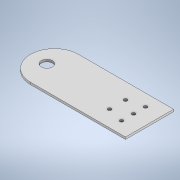
# Autodesk Inventor part: Beslag ekstra håndtag
Saved by Autodesk Inventor 2022 (Build 260153000, 153)
## iProperties
Created: 2022-04-12
Part Number: Beslag ekstra håndtag
Material: Generic
Document SubType Name: Sheet Metal
Designer: Patrick
Density: 1 g/cm^3
Sheet Metal Rule: Default_mm
Appearance: Default
Author: Patrick
Autodesk Inventor part; units mm, degrees
ref_plane "YZ Plane" through (0, 0, 0) normal (1, 0, 0) x (0, 1, 0)
ref_plane "XZ Plane" through (0, 0, 0) normal (0, 1, 0) x (-1, 0, 0)
ref_plane "XY Plane" through (0, 0, 0) normal (0, 0, 1) x (1, 0, 0)
sketch "Sketch2" plane through (0, 0, 0) normal (0, 1, 0) x (-1, 0, 0)
  line L0 (0, 0) -> (109, 0)
  line L1 (109, 0) -> (109, -44)
  line L2 (109, -44) -> (0, -44)
  line L3 (0, -44) -> (0, 0)
  line L4 (44, 0) -> (44, -44) construction
  arc A0 (87, -44) -> (87, 0) centre (87, -22) ccw
  circle A1 centre (94, -22) radius 5.1
  circle A2 centre (29.3333, -14.6667) radius 1.625
  circle A3 centre (29.3333, -29.3333) radius 1.625
  circle A4 centre (14.6667, -11) radius 1.625
  circle A5 centre (14.6667, -22) radius 1.625
  circle A6 centre (14.6667, -33) radius 1.625
  dimension "d36" = 44
  dimension "d37" = 44
  dimension "d38" = 65
  dimension "d41" = 10.2
  dimension "d42" = 22
  dimension "d43" = 15
  dimension "d44" = 14.6667
  dimension "d45" = 14.6667
  dimension "d46" = 14.6667
  dimension "d47" = 11
  dimension "d48" = 11
  dimension "d49" = 11
  dimension "d50" = 11
  dimension "d51" = 3.25
  dimension "d52" = 3.25
  dimension "d53" = 3.25
  dimension "d54" = 3.25
  dimension "d55" = 3.25
  dimension "d56" = 14.6667
  dimension "d57" = 14.6667
  dimension "d58" = 14.6667
  dimension "d59" = 14.6667
  measures "d36" distance between parallel lines of L3 L4
  measures "d37" distance of L2.end L0.start
  measures "d38" distance between parallel lines of L4 L1
  measures "d41" diameter of A1
  measures "d42" distance from line of L2 A1.centre
  measures "d43" distance from line of A1.centre L1
  measures "d44" distance from line of L2 A3.centre
  measures "d45" distance from line of L0 A2.centre
  measures "d46" distance of A2.centre A3.centre
  measures "d47" distance from line of L2 A6.centre
  measures "d48" distance of A5.centre A6.centre
  measures "d49" distance of A5.centre A4.centre
  measures "d50" distance from line of L0 A4.centre
  measures "d51" diameter of A2
  measures "d52" diameter of A3
  measures "d53" diameter of A4
  measures "d54" diameter of A5
  measures "d55" diameter of A6
  measures "d56" distance from line of L4 A3.centre
  measures "d57" distance from line of L4 A2.centre
  measures "d58" distance from line of L3 A6.centre
  measures "d59" distance from line of L3 A4.centre
extrude "Plate3" add sketch "Sketch2" along normal blind 2 contours L0 A0 L2 L3
equation "\"d42\" = 0.5 * d37"
equation "\"d44\" = 0.333333 * d37"
equation "\"d45\" = d44"
equation "\"d47\" = 0.25 * d37"
equation "\"d48\" = d47"
equation "\"d49\" = d47"
equation "\"d52\" = d51"
equation "\"d53\" = d51"
equation "\"d54\" = d51"
equation "\"d55\" = d51"
equation "\"d56\" = 0.333333 * d36"
equation "\"d57\" = d56"
equation "\"d58\" = d46"
equation "\"d59\" = d46"
equation "\"d60\" = Thickness"
equation "\"BendRadius\" = Thickness"
equation "\"BendReliefWidth\" = Thickness"
equation "\"BendReliefDepth\" = 0.5 * Thickness"
equation "\"CornerReliefSize\" = 4 * Thickness"
equation "\"MinimumRemnant\" = 2 * Thickness"
equation "\"TransitionRadius\" = BendRadius"
equation "\"JacobiRadiusSize\" = BendRadius"
equation "\"GapSize\" = Thickness"
equation "\"Thickness\" = 2"
body "Solid3"
